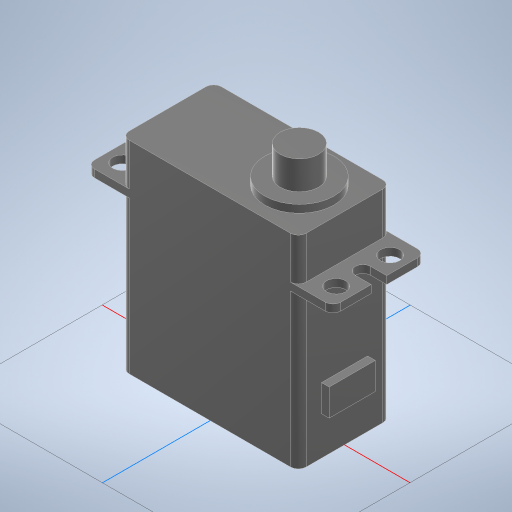
# Autodesk Inventor part: servo_alzrc_ds452mg
Saved by Autodesk Inventor 2023 (Build 270158000, 158)
## iProperties
Created: 2022-06-13
Part Number: servo_alzrc_ds452mg
Material: Thermoplastic Resin
Document SubType Name: Modeling
Designer: dennis
Density: 1.28 g/cm^3
Appearance: Smooth - Black
Author: dennis
Autodesk Inventor part; units mm, degrees
ref_plane "YZ Plane" through (0, 0, 0) normal (1, 0, 0) x (0, 1, 0)
ref_plane "XZ Plane" through (0, 0, 0) normal (0, 1, 0) x (-1, 0, 0)
ref_plane "XY Plane" through (0, 0, 0) normal (0, 0, 1) x (1, 0, 0)
sketch "Sketch1" plane through (0, 0, 0) normal (0, 0, 1) x (1, 0, 0)
  line L0 (-35.5537, 46.3091) -> (69.62, 46.3091) construction
  line L1 (69.62, 46.3091) -> (69.62, -40.915) construction
  line L2 (69.62, -40.915) -> (-35.5537, -40.915) construction
  line L3 (-35.5537, -40.915) -> (-35.5537, 46.3091) construction
  line L4 (-11.5, -3.1187) -> (11.5, -3.1187)
  point P0 (0, 0)
  point P1 (0, 0)
  dimension "d19" = 23
  constraints: 4 end point, 1 horizontal, 2 other
  measures "d19" distance of L4.start L4.end
sketch "Sketch5" plane through (0, 0, 0) normal (0, 1, 0) x (-1, 0, 0)
  line L0 (-51.6883, 69.5392) -> (52.6581, 69.5392) construction
  line L1 (52.6581, 69.5392) -> (52.6581, -16.9988) construction
  line L2 (52.6581, -16.9988) -> (-51.6883, -16.9988) construction
  line L3 (-51.6883, -16.9988) -> (-51.6883, 69.5392) construction
  line L4 (16, 8.395) -> (-16, 8.395)
  circle A0 centre (-5.616, 0) radius 2.5
  circle A1 centre (-5.616, 0) radius 4.5
  circle A2 centre (-13.9015, 3.5026) radius 1.25
  line L5 (-5.616, 0) -> (-20.9236, 0)
  circle A3 centre (-13.9015, -3.5026) radius 1.25
  line L6 (0, 0) -> (0, -9.2667)
  circle A4 centre (13.9015, 3.5026) radius 1.25
  circle A5 centre (13.9015, -3.5026) radius 1.25
  line L7 (13.9015, -3.5026) -> (13.9015, 3.5026)
  arc A6 (13.9015, 1.0292) -> (13.9015, -0.9708) centre (13.9015, 0.0292) ccw
  line L8 (13.9015, -0.9708) -> (16.5074, -0.9708)
  line L9 (16.5074, 1.0292) -> (13.9015, 1.0292)
  line L10 (16.5074, -0.9708) -> (16.5074, 1.0292)
  point P0 (0, 8.395)
  dimension "d30" = 32
  dimension "d57" = 9
  dimension "d58" = 5
  dimension "d63" = 2.5
  dimension "d83" = 2
  dimension "d84" = 1
  constraints: 16 end point, 7 centre point, 3 horizontal, 3 symmetric about line, 2 point on circle, 2 point on line, 2 vertical, 1 coincident, 1 midpoint, 1 perpendicular, 5 other
  measures "d30" distance of L4.start L4.end
  measures "d57" diameter of A1
  measures "d58" diameter of A0
  measures "d63" diameter of A2
  measures "d83" distance of L8.start L9.end
  measures "d84" radius of A6
sketch "Sketch6" plane through (0, 0, 0) normal (0, 1, 0) x (-1, 0, 0)
  line L0 (11.515, 6.0048) -> (11.515, -5.9952)
  line L1 (11.515, 0.0048) -> (-11.485, 0.0048)
  line L2 (11.515, -5.9952) -> (11.515, 6.0048)
  line L3 (-11.485, 6.0048) -> (-11.485, -5.9952)
  line L4 (11.515, -5.9952) -> (-11.485, -5.9952)
  line L5 (-11.485, 6.0048) -> (11.515, 6.0048)
  point P0 (0, 0)
  point P1 (9.3248, 11.448)
  point P2 (-11.485, 0.0048)
  dimension "d42" = 12
  dimension "d43" = 23
  dimension "d44" = 12
  constraints: 12 end point, 2 midpoint, 2 symmetric about line, 2 vertical, 1 horizontal, 1 perpendicular
  measures "d42" distance of L0.start L0.end
  measures "d43" distance of L1.start L1.end
  measures "d44" distance of L3.start L3.end
extrude "Extrusion1" add sketch "Sketch6" along normal blind 26.3
extrude "Extrusion2" add sketch "Sketch5" along normal blind 1 from surface at 26.3 contours A0 | A1
sketch "Sketch7" plane through (-11.515, 0, -5.9952) normal (-1, 0, 0) x (0, 0, 1)
  line L0 (5.9952, 0) -> (5.9952, 19.8)
  line L1 (5.9952, 19.8) -> (5.9952, 20.8)
  line L2 (0, 0) -> (0, 26.3) projected
  line L3 (0, 19.8) -> (12, 19.8)
  line L4 (12, 0) -> (12, 26.3) projected
  line L5 (12, 20.8) -> (0, 20.8)
  line L6 (0, 20.8) -> (0, 19.8)
  dimension "d49" = 19.8
  dimension "d50" = 1
  constraints: 10 end point, 3 point on line, 2 horizontal, 1 perpendicular, 1 vertical
  measures "d49" distance of L0.start L0.end
  measures "d50" distance of L0.end L1.end
extrude "Extrusion3" add sketch "Sketch7" along normal blind 4.5
sketch "Sketch8" plane through (11.485, 0, 6.0048) normal (1, 0, 0) x (0, 0, -1)
  line L0 (6.0048, 0) -> (6.0048, 19.8)
  line L1 (6.0048, 19.8) -> (6.0048, 20.8)
  line L2 (0, 0) -> (0, 26.3) projected
  line L3 (0, 19.7999) -> (12, 19.7999)
  line L4 (12, 20.8) -> (12, 19.8) projected
  line L5 (12, 19.7999) -> (12, 20.8)
  line L6 (12, 20.8) -> (0, 20.8)
  line L7 (0, 20.8) -> (0, 19.7999)
  dimension "d53" = 19.8
  dimension "d54" = 1
  constraints: 10 end point, 3 vertical, 2 perpendicular, 2 point on line, 3 other
  measures "d53" distance of L0.start L0.end
  measures "d54" distance of L0.end L1.end
extrude "Extrusion4" add sketch "Sketch8" along normal blind 4.5
extrude "Extrusion5" add sketch "Sketch5" along normal blind 3.7 from surface at 27.3 contours A0
fillet "Fillet1" radius 1 12 edges at (11.485, 9.8999, 6.0048) (11.485, 9.8999, -5.9952) (-11.515, 9.9, -5.9952) (-11.515, 23.55, -5.9952) (-11.515, 23.55, 6.0048) (-11.515, 9.9, 6.0048) (-16.015, 20.3, 6.0048) (-16.015, 20.3, -5.9952) (11.485, 23.55, -5.9952) (15.985, 20.2999, -5.9952) (15.985, 20.2999, 6.0048) (11.485, 23.55, 6.0048)
extrude "Extrusion6" cut sketch "Sketch5" along normal up to surface (20.8 mm away) contours A2
extrude "Extrusion7" cut sketch "Sketch5" along normal up to surface (20.8 mm away) contours A3
extrude "Extrusion8" cut sketch "Sketch5" along normal up to surface (20.8 mm away) contours A4
extrude "Extrusion9" cut sketch "Sketch5" along normal up to surface (20.8 mm away) contours A5
sketch "Sketch9" plane through (11.485, 0, 5.0048) normal (1, 0, 0) x (0, 0, -1)
  line L0 (10, 26.3) -> (10, 20.8) projected
  line L1 (11, 0) -> (10, 0) projected
  line L2 (10, 26.3) -> (10, 0)
  line L3 (10, 19.7999) -> (10, 0) projected
  line L4 (0, 0) -> (0, 19.7999) projected
  line L5 (5.0048, 0) -> (5.0048, 5)
  line L6 (5.0048, 5) -> (5.0048, 8.5)
  line L7 (5.0048, 5) -> (8.0048, 5)
  line L8 (5.0048, 5) -> (2.0048, 5)
  line L9 (2.0048, 5) -> (2.0048, 8.5)
  line L10 (2.0048, 8.5) -> (8.0048, 8.5)
  line L11 (8.0048, 8.5) -> (8.0048, 5)
  dimension "d76" = 26.3
  dimension "d77" = 5
  dimension "d78" = 3.5
  dimension "d79" = 3
  constraints: 16 end point, 3 vertical, 2 perpendicular, 1 horizontal, 1 point on line, 1 symmetric about line
  measures "d76" distance of L0.start L1.end
  measures "d77" distance of L5.start L5.end
  measures "d78" distance of L5.end L6.end
  measures "d79" distance of L5.end L7.end
extrude "Extrusion10" add sketch "Sketch9" along normal blind 1
extrude "Extrusion11" cut sketch "Sketch5" along normal up to surface (20.8 mm away) contours L9 L10 L8 L7 | L7 A6
mirror "Spiegeln1" about plane through (0, 0, 0) normal (1, 0, 0) of "Extrusion11"
ref_plane "Arbeitsebene1" through (0, 0, 0) normal (1, 0, 0) x (0, 1, 0)
body "Solid1"
